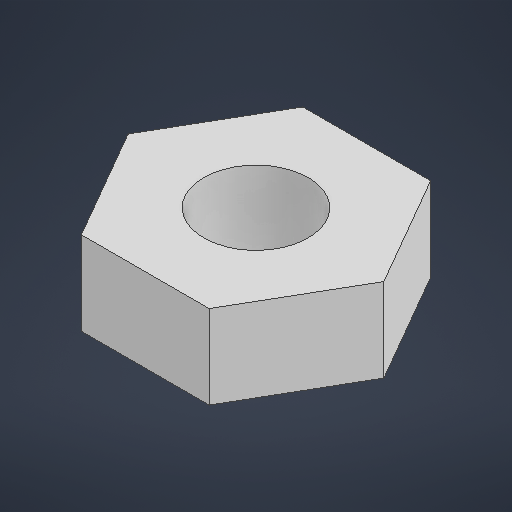
# Autodesk Inventor part: spoolfixer
Saved by Autodesk Inventor 2026.2 (Build 302298010, 298A)
## iProperties
Created: 2026-03-06
Part Number: spoolfixer
Material: Generic
Document SubType Name: Modeling
Designer: Luke
Density: 1 g/cm^3
Appearance: Default
Author: Luke
Autodesk Inventor part; units mm, degrees
ref_plane "YZ Plane" through (0, 0, 0) normal (1, 0, 0) x (0, 1, 0)
ref_plane "XZ Plane" through (0, 0, 0) normal (0, 1, 0) x (-1, 0, 0)
ref_plane "XY Plane" through (0, 0, 0) normal (0, 0, 1) x (1, 0, 0)
sketch "Sketch1" plane through (0, 0, 0) normal (0, 1, 0) x (-1, 0, 0)
  line L0 (-1.53, -2.65) -> (-3.06, 0)
  line L1 (-3.06, 0) -> (-1.53, 2.65)
  line L2 (-1.53, 2.65) -> (1.53, 2.65)
  line L3 (1.53, 2.65) -> (3.06, 0)
  line L4 (3.06, 0) -> (1.53, -2.65)
  line L5 (1.53, -2.65) -> (-1.53, -2.65)
  circle A0 centre (0, 0) radius 1.25
  circle A1 centre (0, 0) radius 2.65 construction
  dimension "d0" = 2.5
  dimension "d3" = 5.3
  constraints: 12 end point, 3 coincident, 2 centre point, 1 horizontal, 1 tangent, 13 other
  measures "d0" diameter of A0
  measures "d3" diameter of A1
extrude "Extrusion1" add sketch "Sketch1" along normal blind 2
body "Solid1"
